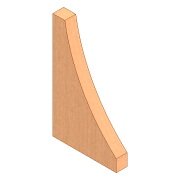
# Autodesk Inventor part: arms
Saved by Autodesk Inventor 2020 (Build 240168000, 168)
## iProperties
Created: 2021-06-24
Part Number: arms
Material: Generic
Document SubType Name: Modeling
Designer: Aidan Lee
Density: 1 g/cm^3
Appearance: Cherry - Natural Low Gloss
Author: Aidan Lee
Autodesk Inventor part; units mm, degrees
ref_plane "YZ Plane" through (0, 0, 0) normal (1, 0, 0) x (0, 1, 0)
ref_plane "XZ Plane" through (0, 0, 0) normal (0, 1, 0) x (-1, 0, 0)
ref_plane "XY Plane" through (0, 0, 0) normal (0, 0, 1) x (1, 0, 0)
sketch "Sketch1" plane through (0, 0, 0) normal (0, 0, 1) x (1, 0, 0)
  line L0 (0, 0) -> (140, 0) construction
  line L1 (140, 0) -> (140, 300) construction
  line L2 (140, 300) -> (0, 300) construction
  line L3 (0, 300) -> (0, 0) construction
  line L4 (70, 308.6686) -> (70, 317.1965) construction
  line L5 (130, 290) -> (130, 293.3347) construction
  line L6 (0, 160.5) -> (-18, 160.5) construction
  line L7 (-18, 160.5) -> (-18, 180.5) construction
  line L8 (-18, 180.5) -> (0, 180.5) construction
  line L9 (0, 180.5) -> (0, 160.5) construction
  line L10 (-16.3067, 150) -> (-26.4998, 150) construction
  circle A0 centre (-9, 170.5) radius 3 construction
  line L11 (-18, 180.5) -> (0, 200.5) construction
  line L12 (0, 139.5) -> (-18, 139.5) construction
  line L13 (-18, 139.5) -> (-18, 119.5) construction
  circle A1 centre (-9, 129.5) radius 3 construction
  line L14 (-18, 119.5) -> (0, 99.5) construction
  line L15 (140, 160.5) -> (158, 160.5) construction
  line L16 (158, 160.5) -> (158, 180.5) construction
  circle A2 centre (149, 170.5) radius 3 construction
  line L17 (158, 180.5) -> (140, 200.5) construction
  line L18 (158, 139.5) -> (158, 119.5) construction
  line L19 (140, 139.5) -> (158, 139.5) construction
  circle A3 centre (149, 129.5) radius 3 construction
  line L20 (158, 119.5) -> (140, 99.5) construction
  line L21 (158, 186) -> (140, 186) construction
  line L22 (140, 186) -> (140, 114) construction
  line L23 (140, 114) -> (158, 114) construction
  line L24 (158, 114) -> (158, 186) construction
  line L25 (158, 156.5) -> (153, 156.5) construction
  line L26 (153, 156.5) -> (153, 143.5) construction
  line L27 (153, 143.5) -> (158, 143.5) construction
  line L28 (158, 143.5) -> (158, 156.5) construction
  line L29 (153, 152) -> (165, 152) construction
  line L30 (165, 152) -> (165, 148) construction
  line L31 (165, 148) -> (153, 148) construction
  line L32 (153, 148) -> (153, 152) construction
  line L33 (158.25, 155.5) -> (159.85, 155.5) construction
  line L34 (159.85, 155.5) -> (159.85, 144.5) construction
  line L35 (159.85, 144.5) -> (158.25, 144.5) construction
  line L36 (158.25, 144.5) -> (158.25, 155.5) construction
  line L37 (160.1, 156.5) -> (165.1, 156.5) construction
  line L38 (165.1, 156.5) -> (165.1, 143.5) construction
  line L39 (165.1, 143.5) -> (160.1, 143.5) construction
  line L40 (160.1, 143.5) -> (160.1, 156.5) construction
  line L41 (160.1, 166.5) -> (160.1, -9)
  line L42 (160.1, 166.5) -> (180.1, 166.5)
  line L43 (160.1, -9) -> (70, -9) construction
  line L44 (160.1, -9) -> (265.1, -9)
  line L45 (265.1, -9) -> (265.1, 11)
  arc A4 (180.1, 166.5) -> (265.1, 11) centre (442.3295, 208.8594) ccw
  point P0 (70, 300)
  point P1 (10, 150)
  point P2 (0, 150)
  point P3 (70, 312.9325)
  point P4 (-21.4032, 150)
  point P5 (-18, 170.5)
  point P6 (-9, 180.5)
  point P7 (153, 150)
  point P8 (140, 150)
  point P9 (153, 150)
  point P10 (158.25, 150)
  dimension "d0" = 140
  dimension "d1" = 300
  dimension "d85" = 18
  dimension "d86" = 20
  dimension "d87" = 10.5
  dimension "d88" = 6
  dimension "d89" = 20
  dimension "racewidth" = 5
  dimension "d110" = 13
  dimension "d111" = 12
  dimension "d112" = 4
  dimension "d113" = 1.6
  dimension "d114" = 5
  dimension "d117" = 11
  dimension "gap" = 0.25
  dimension "d119" = 0.25
  dimension "d120" = 0
  dimension "d121" = 10
  dimension "d122" = 20
  dimension "d123" = 9
  dimension "d124" = 20.1
  dimension "d126" = 105
  dimension "d127" = 20
  dimension "d128" = 0.1
  dimension "d129" = 175.5
  dimension "d132" = 16.5
  dimension "d147" = 90.1
  dimension "d148" = 2.1
  constraints: 92 end point, 15 symmetric about line, 14 parallel, 11 horizontal, 10 midpoint, 7 horizontal alignment, 7 perpendicular, 5 centre point, 4 point on line, 4 vertical, 3 vertical alignment, 2 collinear, 2 point on circle, 1 coincident, 3 other
  measures "d0" distance of L0.start L0.end
  measures "d1" distance of L2.end L0.start
  measures "d85" distance of L7.end L8.end
  measures "d86" distance of L6.end L7.end
  measures "d87" distance between parallel lines of L6 L10
  measures "d88" diameter of A0
  measures "d89" vertical distance of L7.end L11.end
  measures "racewidth" distance of L25.start L25.end
  measures "d110" distance of L25.end L26.end
  measures "d111" distance of L30.end L31.end
  measures "d112" distance of L31.end L29.start
  measures "d113" distance of L33.start L33.end
  measures "d114" distance of L37.start L37.end
  measures "d117" distance of L33.end L34.end
  measures "gap" distance between parallel lines of L36 L24
  measures "d119" distance between parallel lines of L34 L40
  measures "d120" distance between parallel lines of L26 L32
  measures "d121" distance from line of L41.start L37
  measures "d122" distance of L41.start L42.end
  measures "d123" distance between parallel lines of L0 L43
  measures "d124" distance between parallel lines of L41 L1
  measures "d126" distance of L41.end L44.end
  measures "d127" distance of L44.end L45.end
  measures "d128" distance between parallel lines of L30 L38
  measures "d129" distance of L41.start L41.end
  measures "d132" distance from line of L42 point (158.25, 150)
  measures "d147" distance between parallel lines of L4 L41
  measures "d148" distance between parallel lines of L24 L41
extrude "Extrusion1" add sketch "Sketch1" along normal blind 18
sketch "Sketch2" plane through (160.1, -9, 0) normal (-1, 0, 0) x (0, 0, 1)
  circle A0 centre (9, 157.5) radius 6.5
  line L0 (0, 175.5) -> (18, 175.5) projected
  point P0 (0, 9)
  point P1 (9, 175.5)
  dimension "bearingdiameter" = 13
  dimension "d134" = 18
  constraints: 1 centre point, 1 midpoint, 1 vertical alignment
  measures "bearingdiameter" diameter of A0
  measures "d134" distance from line of L0 A0.centre
extrude "Extrusion2" cut sketch "Sketch2" against normal blind 5
sketch "Sketch3" plane through (160.1, -9, 0) normal (0, -1, 0) x (1, 0, 0)
  circle A0 centre (22.5, 9) radius 0.75
  line L0 (0, 0) -> (0, 18) projected
  line L1 (0, 0) -> (105, 0) projected
  circle A1 centre (52.5, 9) radius 0.75
  circle A2 centre (82.5, 9) radius 0.75
  point P0 (-160.1, 0)
  point P1 (0, 9)
  point P2 (52.5, 0)
  dimension "d137" = 1.5
  dimension "d140" = 30
  constraints: 3 centre point, 2 midpoint, 1 horizontal, 1 horizontal alignment, 1 vertical alignment, 4 other
  measures "d137" diameter of A0
  measures "d140" distance of A0.centre A1.centre
extrude "Extrusion3" cut sketch "Sketch3" against normal blind 22
body "Solid1"
